Autodesk Fusion 360 part; units mm, degrees
note: some values were not read from the file. Set by a fixed rule: which sketch regions a step uses.
(part 2 of 3)
sketch "Sketch3" plane through (0, 0, -2) normal (0, 0, -1) x (1, 0, 0)
  line L0 (37.09, -0.4341) -> (37.09, -14.4986)
  arc A0 (32.09, -19.4986) -> (37.09, -14.4986) centre (32.09, -14.4986) ccw
  line L1 (32.09, -19.4986) -> (5.9194, -19.4986)
  arc A1 (0.9194, -14.4986) -> (5.9194, -19.4986) centre (5.9194, -14.4986) ccw
  line L2 (0.9194, -14.4986) -> (0.9194, -0.4341)
  line L3 (0.9194, -0.4341) -> (0.0951, -0.4341)
  line L4 (0.0951, -0.4341) -> (0.0951, -148.071)
  line L5 (0.0951, -148.071) -> (76.2953, -148.071)
  line L6 (76.2953, -148.071) -> (76.2953, -75.8337)
  line L7 (76.2953, -75.8337) -> (61.902, -75.8337)
  arc A2 (56.902, -70.8337) -> (61.902, -75.8337) centre (61.902, -70.8337) ccw
  line L8 (56.902, -70.8337) -> (56.902, -44.1838)
  arc A3 (61.902, -39.1838) -> (56.902, -44.1838) centre (61.902, -44.1838) ccw
  line L9 (61.902, -39.1838) -> (76.2953, -39.1838)
  line L10 (76.2953, -39.1838) -> (76.2953, -36.6991)
  line L11 (76.2953, -36.6991) -> (61.902, -36.6991)
  arc A4 (56.902, -31.6991) -> (61.902, -36.6991) centre (61.902, -31.6991) ccw
  line L12 (56.902, -31.6991) -> (56.902, -6.8092)
  arc A5 (61.902, -1.8092) -> (56.902, -6.8092) centre (61.902, -6.8092) ccw
  line L13 (61.902, -1.8092) -> (76.2953, -1.8092)
  line L14 (76.2953, -1.8092) -> (76.2953, -0.4341)
  line L15 (76.2953, -0.4341) -> (37.09, -0.4341)
  line L16 (40.7197, -3.5609) -> (40.7197, -1.96)
  line L17 (40.7197, -1.96) -> (54.719, -1.96)
  line L18 (54.719, -1.96) -> (54.719, -3.5609)
  line L19 (54.719, -3.5609) -> (55.5198, -3.5609)
  line L20 (55.5198, -3.5609) -> (55.5198, -16.3601)
  line L21 (55.5198, -16.3601) -> (54.719, -16.3601)
  line L22 (54.719, -16.3601) -> (54.719, -17.9595)
  line L23 (54.719, -17.9595) -> (40.7197, -17.9595)
  line L24 (40.7197, -17.9595) -> (40.7197, -16.3601)
  line L25 (40.7197, -16.3601) -> (39.9189, -16.3601)
  line L26 (39.9189, -16.3601) -> (39.9189, -3.5609)
  line L27 (39.9189, -3.5609) -> (40.7197, -3.5609)
  line L28 (2.6197, -79.7609) -> (2.6197, -78.1602)
  line L29 (2.6197, -78.1602) -> (16.6192, -78.1602)
  line L30 (16.6192, -78.1602) -> (16.6192, -79.7609)
  line L31 (16.6192, -79.7609) -> (17.4198, -79.7609)
  line L32 (17.4198, -79.7609) -> (17.4198, -92.5601)
  line L33 (17.4198, -92.5601) -> (16.6192, -92.5601)
  line L34 (16.6192, -92.5601) -> (16.6192, -94.1594)
  line L35 (16.6192, -94.1594) -> (2.6196, -94.1594)
  line L36 (2.6197, -94.1594) -> (2.6197, -92.5601)
  line L37 (2.6197, -92.5601) -> (1.819, -92.5601)
  line L38 (1.819, -92.5601) -> (1.819, -79.7609)
  line L39 (1.819, -79.7609) -> (2.6197, -79.7609)
  line L40 (21.6697, -22.6109) -> (21.6697, -21.01)
  line L41 (21.6697, -21.01) -> (35.669, -21.01)
  line L42 (35.669, -21.01) -> (35.669, -22.6109)
  line L43 (35.669, -22.6109) -> (36.4698, -22.6109)
  line L44 (36.4698, -22.6109) -> (36.4698, -35.4101)
  line L45 (36.4698, -35.4101) -> (35.669, -35.4101)
  line L46 (35.669, -35.4101) -> (35.669, -37.0094)
  line L47 (35.669, -37.0094) -> (21.6697, -37.0094)
  line L48 (21.6697, -37.0094) -> (21.6697, -35.4101)
  line L49 (21.6697, -35.4101) -> (20.869, -35.4101)
  line L50 (20.869, -35.4101) -> (20.869, -22.6109)
  line L51 (20.869, -22.6109) -> (21.6697, -22.6109)
  line L52 (40.7197, -41.6609) -> (40.7197, -40.0602)
  line L53 (40.7197, -40.0602) -> (54.719, -40.0602)
  line L54 (54.719, -40.0602) -> (54.719, -41.6609)
  line L55 (54.719, -41.6609) -> (55.5198, -41.6609)
  line L56 (55.5198, -41.6609) -> (55.5198, -54.4601)
  line L57 (55.5198, -54.4601) -> (54.719, -54.4601)
  line L58 (54.719, -54.4601) -> (54.719, -56.0594)
  line L59 (54.719, -56.0594) -> (40.7197, -56.0594)
  line L60 (40.7197, -56.0594) -> (40.7197, -54.4601)
  line L61 (40.7197, -54.4601) -> (39.9189, -54.4601)
  line L62 (39.9189, -54.4601) -> (39.9189, -41.6609)
  line L63 (39.9189, -41.6609) -> (40.7197, -41.6609)
  line L64 (40.7197, -22.6109) -> (40.7197, -21.01)
  line L65 (40.7197, -21.01) -> (54.719, -21.01)
  line L66 (54.719, -21.01) -> (54.719, -22.6109)
  line L67 (54.719, -22.6109) -> (55.5198, -22.6109)
  line L68 (55.5198, -22.6109) -> (55.5198, -35.4101)
  line L69 (55.5198, -35.4101) -> (54.719, -35.4101)
  line L70 (54.719, -35.4101) -> (54.719, -37.0094)
  line L71 (54.719, -37.0094) -> (40.7197, -37.0094)
  line L72 (40.7197, -37.0094) -> (40.7197, -35.4101)
  line L73 (40.7197, -35.4101) -> (39.9189, -35.4101)
  line L74 (39.9189, -35.4101) -> (39.9189, -22.6109)
  line L75 (39.9189, -22.6109) -> (40.7197, -22.6109)
  line L76 (40.7197, -60.7109) -> (40.7197, -59.1102)
  line L77 (40.7197, -59.1102) -> (54.719, -59.1102)
  line L78 (54.719, -59.1102) -> (54.719, -60.7109)
  line L79 (54.719, -60.7109) -> (55.5198, -60.7109)
  line L80 (55.5198, -60.7109) -> (55.5198, -73.5101)
  line L81 (55.5198, -73.5101) -> (54.719, -73.5101)
  line L82 (54.719, -73.5101) -> (54.719, -75.1094)
  line L83 (54.719, -75.1094) -> (40.7197, -75.1094)
  line L84 (40.7197, -75.1094) -> (40.7197, -73.5101)
  line L85 (40.7197, -73.5101) -> (39.9189, -73.5101)
  line L86 (39.9189, -73.5101) -> (39.9189, -60.7109)
  line L87 (39.9189, -60.7109) -> (40.7197, -60.7109)
  line L88 (21.6697, -41.6609) -> (21.6697, -40.0602)
  line L89 (21.6697, -40.0602) -> (35.669, -40.0602)
  line L90 (35.669, -40.0602) -> (35.669, -41.6609)
  line L91 (35.669, -41.6609) -> (36.4698, -41.6609)
  line L92 (36.4698, -41.6609) -> (36.4698, -54.4601)
  line L93 (36.4698, -54.4601) -> (35.669, -54.4601)
  line L94 (35.669, -54.4601) -> (35.669, -56.0594)
  line L95 (35.669, -56.0594) -> (21.6697, -56.0594)
  line L96 (21.6697, -56.0594) -> (21.6697, -54.4601)
  line L97 (21.6697, -54.4601) -> (20.869, -54.4601)
  line L98 (20.869, -54.4601) -> (20.869, -41.6609)
  line L99 (20.869, -41.6609) -> (21.6697, -41.6609)
  line L100 (2.6197, -41.6609) -> (2.6197, -40.0602)
  line L101 (2.6197, -40.0602) -> (16.6192, -40.0602)
  line L102 (16.6192, -40.0602) -> (16.6192, -41.6609)
  line L103 (16.6192, -41.6609) -> (17.4198, -41.6609)
  line L104 (17.4198, -41.6609) -> (17.4198, -54.4601)
  line L105 (17.4198, -54.4601) -> (16.6192, -54.4601)
  line L106 (16.6192, -54.4601) -> (16.6192, -56.0594)
  line L107 (16.6192, -56.0594) -> (2.6196, -56.0594)
  line L108 (2.6197, -56.0594) -> (2.6197, -54.4601)
  line L109 (2.6197, -54.4601) -> (1.819, -54.4601)
  line L110 (1.819, -54.4601) -> (1.819, -41.6609)
  line L111 (1.819, -41.6609) -> (2.6197, -41.6609)
  line L112 (2.6197, -22.6109) -> (2.6197, -21.01)
  line L113 (2.6197, -21.01) -> (16.6192, -21.01)
  line L114 (16.6192, -21.01) -> (16.6192, -22.6109)
  line L115 (16.6192, -22.6109) -> (17.4198, -22.6109)
  line L116 (17.4198, -22.6109) -> (17.4198, -35.4101)
  line L117 (17.4198, -35.4101) -> (16.6192, -35.4101)
  line L118 (16.6192, -35.4101) -> (16.6192, -37.0094)
  line L119 (16.6192, -37.0094) -> (2.6196, -37.0094)
  line L120 (2.6197, -37.0094) -> (2.6197, -35.4101)
  line L121 (2.6197, -35.4101) -> (1.819, -35.4101)
  line L122 (1.819, -35.4101) -> (1.819, -22.6109)
  line L123 (1.819, -22.6109) -> (2.6197, -22.6109)
  line L124 (40.7197, -79.7609) -> (40.7197, -78.1602)
  line L125 (40.7197, -78.1602) -> (54.719, -78.1602)
  line L126 (54.719, -78.1602) -> (54.719, -79.7609)
  line L127 (54.719, -79.7609) -> (55.5198, -79.7609)
  line L128 (55.5198, -79.7609) -> (55.5198, -92.5601)
  line L129 (55.5198, -92.5601) -> (54.719, -92.5601)
  line L130 (54.719, -92.5601) -> (54.719, -94.1594)
  line L131 (54.719, -94.1594) -> (40.7197, -94.1594)
  line L132 (40.7197, -94.1594) -> (40.7197, -92.5601)
  line L133 (40.7197, -92.5601) -> (39.9189, -92.5601)
  line L134 (39.9189, -92.5601) -> (39.9189, -79.7609)
  line L135 (39.9189, -79.7609) -> (40.7197, -79.7609)
  line L136 (59.7697, -79.7609) -> (59.7697, -78.1602)
  line L137 (59.7697, -78.1602) -> (73.769, -78.1602)
  line L138 (73.769, -78.1602) -> (73.769, -79.7609)
  line L139 (73.769, -79.7609) -> (74.5698, -79.7609)
  line L140 (74.5698, -79.7609) -> (74.5698, -92.5601)
  line L141 (74.5698, -92.5601) -> (73.769, -92.5601)
  line L142 (73.769, -92.5601) -> (73.769, -94.1594)
  line L143 (73.769, -94.1594) -> (59.7697, -94.1594)
  line L144 (59.7697, -94.1594) -> (59.7697, -92.5601)
  line L145 (59.7697, -92.5601) -> (58.9689, -92.5601)
  line L146 (58.9689, -92.5601) -> (58.9689, -79.7609)
  line L147 (58.9689, -79.7609) -> (59.7697, -79.7609)
  line L148 (2.6197, -60.7109) -> (2.6197, -59.1102)
  line L149 (2.6197, -59.1102) -> (16.6192, -59.1102)
  line L150 (16.6192, -59.1102) -> (16.6192, -60.7109)
  line L151 (16.6192, -60.7109) -> (17.4198, -60.7109)
  line L152 (17.4198, -60.7109) -> (17.4198, -73.5101)
  line L153 (17.4198, -73.5101) -> (16.6192, -73.5101)
  line L154 (16.6192, -73.5101) -> (16.6192, -75.1094)
  line L155 (16.6192, -75.1094) -> (2.6196, -75.1094)
  line L156 (2.6197, -75.1094) -> (2.6197, -73.5101)
  line L157 (2.6197, -73.5101) -> (1.819, -73.5101)
  line L158 (1.819, -73.5101) -> (1.819, -60.7109)
  line L159 (1.819, -60.7109) -> (2.6197, -60.7109)
  line L160 (59.7697, -117.861) -> (59.7697, -116.26)
  line L161 (59.7697, -116.26) -> (73.769, -116.26)
  line L162 (73.769, -116.26) -> (73.769, -117.861)
  line L163 (73.769, -117.861) -> (74.5698, -117.861)
  line L164 (74.5698, -117.861) -> (74.5698, -130.66)
  line L165 (74.5698, -130.66) -> (73.769, -130.66)
  line L166 (73.769, -130.66) -> (73.769, -132.259)
  line L167 (73.769, -132.259) -> (59.7697, -132.259)
  line L168 (59.7697, -132.259) -> (59.7697, -130.66)
  line L169 (59.7697, -130.66) -> (58.9689, -130.66)
  line L170 (58.9689, -130.66) -> (58.9689, -117.861)
  line L171 (58.9689, -117.861) -> (59.7697, -117.861)
  line L172 (21.6697, -79.7609) -> (21.6697, -78.1602)
  line L173 (21.6697, -78.1602) -> (35.669, -78.1602)
  line L174 (35.669, -78.1602) -> (35.669, -79.7609)
  line L175 (35.669, -79.7609) -> (36.4698, -79.7609)
  line L176 (36.4698, -79.7609) -> (36.4698, -92.5601)
  line L177 (36.4698, -92.5601) -> (35.669, -92.5601)
  line L178 (35.669, -92.5601) -> (35.669, -94.1594)
  line L179 (35.669, -94.1594) -> (21.6697, -94.1594)
  line L180 (21.6697, -94.1594) -> (21.6697, -92.5601)
  line L181 (21.6697, -92.5601) -> (20.869, -92.5601)
  line L182 (20.869, -92.5601) -> (20.869, -79.7609)
  line L183 (20.869, -79.7609) -> (21.6697, -79.7609)
  line L184 (21.6697, -60.7109) -> (21.6697, -59.1102)
  line L185 (21.6697, -59.1102) -> (35.669, -59.1102)
  line L186 (35.669, -59.1102) -> (35.669, -60.7109)
  line L187 (35.669, -60.7109) -> (36.4698, -60.7109)
  line L188 (36.4698, -60.7109) -> (36.4698, -73.5101)
  line L189 (36.4698, -73.5101) -> (35.669, -73.5101)
  line L190 (35.669, -73.5101) -> (35.669, -75.1094)
  line L191 (35.669, -75.1094) -> (21.6697, -75.1094)
  line L192 (21.6697, -75.1094) -> (21.6697, -73.5101)
  line L193 (21.6697, -73.5101) -> (20.869, -73.5101)
  line L194 (20.869, -73.5101) -> (20.869, -60.7109)
  line L195 (20.869, -60.7109) -> (21.6697, -60.7109)
  line L196 (47.7193, -17.9595) -> (47.7193, -1.96)
  line L197 (55.5198, -9.9605) -> (39.9189, -9.9605)
  line L198 (76.2953, -0.4341) -> (76.2953, 14.2999)
  line L199 (0.0951, -0.4341) -> (0.0951, 14.2999)
  line L200 (0.0951, 14.2999) -> (76.2953, 14.2999)
  line L201 (0.0951, -148.071) -> (0.0951, -158.6)
  line L202 (76.2953, -148.071) -> (76.2953, -158.6)
  line L203 (58.9689, -124.2605) -> (74.5698, -124.2605)
  line L204 (76.2953, -158.6) -> (76.2953, -163.6)
  line L205 (0.0951, -158.6) -> (0.0951, -163.6)
  line L206 (0.0951, -163.6) -> (76.2953, -163.6)
  line L207 (37.09, -0.4341) -> (0.0951, -0.4341)
  dimension "d38" = 14.734
  dimension "d39" = 14.734
  dimension "d42" = 5
  dimension "d43" = 5
  dimension "d44" = 177.8999
  constraint midpoint L23 L196.start
  constraint midpoint L17 L196.end
  constraint midpoint L20 L197.start
  constraint midpoint L26 L197.end
  constraint coincident L14.end L15.start
  constraint perpendicular L15 L198
  constraint coincident L3.end L4.start
  constraint perpendicular L3 L199
  constraint coincident L4.end L5.start
  constraint perpendicular L5 L201
  constraint coincident L5.end L6.start
  constraint perpendicular L5 L202
  constraint midpoint L170 L203.start
  constraint midpoint L164 L203.end
  constraint coincident L0.start L15.end
  measures "d38" distance of L14.end L198.end
  measures "d39" distance of L3.end L199.end
  measures "d42" distance of L202.end L204.end
  measures "d43" distance of L201.end L205.end
  measures "d44" distance of L200 L206
extrude "Extrude19" add sketch "Sketch3" against normal blind 3 contours L3 L15 L198 L199 L200 L207 | L5 L201 L202 L204 L205 L206 bodies 1 2
sketch "Sketch4" plane through (0, 0, -2) normal (0, 0, -1) x (1, 0, 0)
  line L0 (37.09, -0.4341) -> (37.09, -14.4986)
  arc A0 (32.09, -19.4986) -> (37.09, -14.4986) centre (32.09, -14.4986) ccw
  line L1 (32.09, -19.4986) -> (5.9194, -19.4986)
  arc A1 (0.9194, -14.4986) -> (5.9194, -19.4986) centre (5.9194, -14.4986) ccw
  line L2 (0.9194, -14.4986) -> (0.9194, -0.4341)
  line L3 (0.9194, -0.4341) -> (37.09, -0.4341)
  line L4 (76.2953, -1.8092) -> (76.2953, 14.2999)
  line L5 (76.2953, 14.2999) -> (0.0951, 14.2999)
  line L6 (0.0951, 14.2999) -> (0.0951, -163.6)
  line L7 (0.0951, -163.6) -> (76.2953, -163.6)
  line L8 (76.2953, -163.6) -> (76.2953, -75.8337)
  line L9 (76.2953, -75.8337) -> (61.902, -75.8337)
  arc A2 (56.902, -70.8337) -> (61.902, -75.8337) centre (61.902, -70.8337) ccw
  line L10 (56.902, -70.8337) -> (56.902, -44.1838)
  arc A3 (61.902, -39.1838) -> (56.902, -44.1838) centre (61.902, -44.1838) ccw
  line L11 (61.902, -39.1838) -> (76.2953, -39.1838)
  line L12 (76.2953, -39.1838) -> (76.2953, -36.6991)
  line L13 (76.2953, -36.6991) -> (61.902, -36.6991)
  arc A4 (56.902, -31.6991) -> (61.902, -36.6991) centre (61.902, -31.6991) ccw
  line L14 (56.902, -31.6991) -> (56.902, -6.8092)
  arc A5 (61.902, -1.8092) -> (56.902, -6.8092) centre (61.902, -6.8092) ccw
  line L15 (61.902, -1.8092) -> (76.2953, -1.8092)
  line L16 (40.7197, -3.5609) -> (40.7197, -1.96)
  line L17 (40.7197, -1.96) -> (54.719, -1.96)
  line L18 (54.719, -1.96) -> (54.719, -3.5609)
  line L19 (54.719, -3.5609) -> (55.5198, -3.5609)
  line L20 (55.5198, -3.5609) -> (55.5198, -16.3601)
  line L21 (55.5198, -16.3601) -> (54.719, -16.3601)
  line L22 (54.719, -16.3601) -> (54.719, -17.9595)
  line L23 (54.719, -17.9595) -> (40.7197, -17.9595)
  line L24 (40.7197, -17.9595) -> (40.7197, -16.3601)
  line L25 (40.7197, -16.3601) -> (39.9189, -16.3601)
  line L26 (39.9189, -16.3601) -> (39.9189, -3.5609)
  line L27 (39.9189, -3.5609) -> (40.7197, -3.5609)
  line L28 (2.6197, -79.7609) -> (2.6197, -78.1602)
  line L29 (2.6197, -78.1602) -> (16.6192, -78.1602)
  line L30 (16.6192, -78.1602) -> (16.6192, -79.7609)
  line L31 (16.6192, -79.7609) -> (17.4198, -79.7609)
  line L32 (17.4198, -79.7609) -> (17.4198, -92.5601)
  line L33 (17.4198, -92.5601) -> (16.6192, -92.5601)
  line L34 (16.6192, -92.5601) -> (16.6192, -94.1594)
  line L35 (16.6192, -94.1594) -> (2.6196, -94.1594)
  line L36 (2.6197, -94.1594) -> (2.6197, -92.5601)
  line L37 (2.6197, -92.5601) -> (1.819, -92.5601)
  line L38 (1.819, -92.5601) -> (1.819, -79.7609)
  line L39 (1.819, -79.7609) -> (2.6197, -79.7609)
  line L40 (21.6697, -22.6109) -> (21.6697, -21.01)
  line L41 (21.6697, -21.01) -> (35.669, -21.01)
  line L42 (35.669, -21.01) -> (35.669, -22.6109)
  line L43 (35.669, -22.6109) -> (36.4698, -22.6109)
  line L44 (36.4698, -22.6109) -> (36.4698, -35.4101)
  line L45 (36.4698, -35.4101) -> (35.669, -35.4101)
  line L46 (35.669, -35.4101) -> (35.669, -37.0094)
  line L47 (35.669, -37.0094) -> (21.6697, -37.0094)
  line L48 (21.6697, -37.0094) -> (21.6697, -35.4101)
  line L49 (21.6697, -35.4101) -> (20.869, -35.4101)
  line L50 (20.869, -35.4101) -> (20.869, -22.6109)
  line L51 (20.869, -22.6109) -> (21.6697, -22.6109)
  line L52 (40.7197, -41.6609) -> (40.7197, -40.0602)
  line L53 (40.7197, -40.0602) -> (54.719, -40.0602)
  line L54 (54.719, -40.0602) -> (54.719, -41.6609)
  line L55 (54.719, -41.6609) -> (55.5198, -41.6609)
  line L56 (55.5198, -41.6609) -> (55.5198, -54.4601)
  line L57 (55.5198, -54.4601) -> (54.719, -54.4601)
  line L58 (54.719, -54.4601) -> (54.719, -56.0594)
  line L59 (54.719, -56.0594) -> (40.7197, -56.0594)
  line L60 (40.7197, -56.0594) -> (40.7197, -54.4601)
  line L61 (40.7197, -54.4601) -> (39.9189, -54.4601)
  line L62 (39.9189, -54.4601) -> (39.9189, -41.6609)
  line L63 (39.9189, -41.6609) -> (40.7197, -41.6609)
  line L64 (40.7197, -22.6109) -> (40.7197, -21.01)
  line L65 (40.7197, -21.01) -> (54.719, -21.01)
  line L66 (54.719, -21.01) -> (54.719, -22.6109)
  line L67 (54.719, -22.6109) -> (55.5198, -22.6109)
  line L68 (55.5198, -22.6109) -> (55.5198, -35.4101)
  line L69 (55.5198, -35.4101) -> (54.719, -35.4101)
  line L70 (54.719, -35.4101) -> (54.719, -37.0094)
  line L71 (54.719, -37.0094) -> (40.7197, -37.0094)
  line L72 (40.7197, -37.0094) -> (40.7197, -35.4101)
  line L73 (40.7197, -35.4101) -> (39.9189, -35.4101)
  line L74 (39.9189, -35.4101) -> (39.9189, -22.6109)
  line L75 (39.9189, -22.6109) -> (40.7197, -22.6109)
  line L76 (40.7197, -60.7109) -> (40.7197, -59.1102)
  line L77 (40.7197, -59.1102) -> (54.719, -59.1102)
  line L78 (54.719, -59.1102) -> (54.719, -60.7109)
  line L79 (54.719, -60.7109) -> (55.5198, -60.7109)
  line L80 (55.5198, -60.7109) -> (55.5198, -73.5101)
  line L81 (55.5198, -73.5101) -> (54.719, -73.5101)
  line L82 (54.719, -73.5101) -> (54.719, -75.1094)
  line L83 (54.719, -75.1094) -> (40.7197, -75.1094)
  line L84 (40.7197, -75.1094) -> (40.7197, -73.5101)
  line L85 (40.7197, -73.5101) -> (39.9189, -73.5101)
  line L86 (39.9189, -73.5101) -> (39.9189, -60.7109)
  line L87 (39.9189, -60.7109) -> (40.7197, -60.7109)
  line L88 (21.6697, -41.6609) -> (21.6697, -40.0602)
  line L89 (21.6697, -40.0602) -> (35.669, -40.0602)
  line L90 (35.669, -40.0602) -> (35.669, -41.6609)
  line L91 (35.669, -41.6609) -> (36.4698, -41.6609)
  line L92 (36.4698, -41.6609) -> (36.4698, -54.4601)
  line L93 (36.4698, -54.4601) -> (35.669, -54.4601)
  line L94 (35.669, -54.4601) -> (35.669, -56.0594)
  line L95 (35.669, -56.0594) -> (21.6697, -56.0594)
  line L96 (21.6697, -56.0594) -> (21.6697, -54.4601)
  line L97 (21.6697, -54.4601) -> (20.869, -54.4601)
  line L98 (20.869, -54.4601) -> (20.869, -41.6609)
  line L99 (20.869, -41.6609) -> (21.6697, -41.6609)
  line L100 (2.6197, -41.6609) -> (2.6197, -40.0602)
  line L101 (2.6197, -40.0602) -> (16.6192, -40.0602)
  line L102 (16.6192, -40.0602) -> (16.6192, -41.6609)
  line L103 (16.6192, -41.6609) -> (17.4198, -41.6609)
  line L104 (17.4198, -41.6609) -> (17.4198, -54.4601)
  line L105 (17.4198, -54.4601) -> (16.6192, -54.4601)
  line L106 (16.6192, -54.4601) -> (16.6192, -56.0594)
  line L107 (16.6192, -56.0594) -> (2.6196, -56.0594)
  line L108 (2.6197, -56.0594) -> (2.6197, -54.4601)
  line L109 (2.6197, -54.4601) -> (1.819, -54.4601)
  line L110 (1.819, -54.4601) -> (1.819, -41.6609)
  line L111 (1.819, -41.6609) -> (2.6197, -41.6609)
  line L112 (2.6197, -22.6109) -> (2.6197, -21.01)
  line L113 (2.6197, -21.01) -> (16.6192, -21.01)
  line L114 (16.6192, -21.01) -> (16.6192, -22.6109)
  line L115 (16.6192, -22.6109) -> (17.4198, -22.6109)
  line L116 (17.4198, -22.6109) -> (17.4198, -35.4101)
  line L117 (17.4198, -35.4101) -> (16.6192, -35.4101)
  line L118 (16.6192, -35.4101) -> (16.6192, -37.0094)
  line L119 (16.6192, -37.0094) -> (2.6196, -37.0094)
  line L120 (2.6197, -37.0094) -> (2.6197, -35.4101)
  line L121 (2.6197, -35.4101) -> (1.819, -35.4101)
  line L122 (1.819, -35.4101) -> (1.819, -22.6109)
  line L123 (1.819, -22.6109) -> (2.6197, -22.6109)
  line L124 (40.7197, -79.7609) -> (40.7197, -78.1602)
  line L125 (40.7197, -78.1602) -> (54.719, -78.1602)
  line L126 (54.719, -78.1602) -> (54.719, -79.7609)
  line L127 (54.719, -79.7609) -> (55.5198, -79.7609)
  line L128 (55.5198, -79.7609) -> (55.5198, -92.5601)
  line L129 (55.5198, -92.5601) -> (54.719, -92.5601)
  line L130 (54.719, -92.5601) -> (54.719, -94.1594)
  line L131 (54.719, -94.1594) -> (40.7197, -94.1594)
  line L132 (40.7197, -94.1594) -> (40.7197, -92.5601)
  line L133 (40.7197, -92.5601) -> (39.9189, -92.5601)
  line L134 (39.9189, -92.5601) -> (39.9189, -79.7609)
  line L135 (39.9189, -79.7609) -> (40.7197, -79.7609)
  line L136 (59.7697, -79.7609) -> (59.7697, -78.1602)
  line L137 (59.7697, -78.1602) -> (73.769, -78.1602)
  line L138 (73.769, -78.1602) -> (73.769, -79.7609)
  line L139 (73.769, -79.7609) -> (74.5698, -79.7609)
  line L140 (74.5698, -79.7609) -> (74.5698, -92.5601)
  line L141 (74.5698, -92.5601) -> (73.769, -92.5601)
  line L142 (73.769, -92.5601) -> (73.769, -94.1594)
  line L143 (73.769, -94.1594) -> (59.7697, -94.1594)
  line L144 (59.7697, -94.1594) -> (59.7697, -92.5601)
  line L145 (59.7697, -92.5601) -> (58.9689, -92.5601)
  line L146 (58.9689, -92.5601) -> (58.9689, -79.7609)
  line L147 (58.9689, -79.7609) -> (59.7697, -79.7609)
  line L148 (2.6197, -60.7109) -> (2.6197, -59.1102)
  line L149 (2.6197, -59.1102) -> (16.6192, -59.1102)
  line L150 (16.6192, -59.1102) -> (16.6192, -60.7109)
  line L151 (16.6192, -60.7109) -> (17.4198, -60.7109)
  line L152 (17.4198, -60.7109) -> (17.4198, -73.5101)
  line L153 (17.4198, -73.5101) -> (16.6192, -73.5101)
  line L154 (16.6192, -73.5101) -> (16.6192, -75.1094)
  line L155 (16.6192, -75.1094) -> (2.6196, -75.1094)
  line L156 (2.6197, -75.1094) -> (2.6197, -73.5101)
  line L157 (2.6197, -73.5101) -> (1.819, -73.5101)
  line L158 (1.819, -73.5101) -> (1.819, -60.7109)
  line L159 (1.819, -60.7109) -> (2.6197, -60.7109)
  line L160 (59.7697, -117.861) -> (59.7697, -116.26)
  line L161 (59.7697, -116.26) -> (73.769, -116.26)
  line L162 (73.769, -116.26) -> (73.769, -117.861)
  line L163 (73.769, -117.861) -> (74.5698, -117.861)
  line L164 (74.5698, -117.861) -> (74.5698, -130.66)
  line L165 (74.5698, -130.66) -> (73.769, -130.66)
  line L166 (73.769, -130.66) -> (73.769, -132.259)
  line L167 (73.769, -132.259) -> (59.7697, -132.259)
  line L168 (59.7697, -132.259) -> (59.7697, -130.66)
  line L169 (59.7697, -130.66) -> (58.9689, -130.66)
  line L170 (58.9689, -130.66) -> (58.9689, -117.861)
  line L171 (58.9689, -117.861) -> (59.7697, -117.861)
  line L172 (21.6697, -79.7609) -> (21.6697, -78.1602)
  line L173 (21.6697, -78.1602) -> (35.669, -78.1602)
  line L174 (35.669, -78.1602) -> (35.669, -79.7609)
  line L175 (35.669, -79.7609) -> (36.4698, -79.7609)
  line L176 (36.4698, -79.7609) -> (36.4698, -92.5601)
  line L177 (36.4698, -92.5601) -> (35.669, -92.5601)
  line L178 (35.669, -92.5601) -> (35.669, -94.1594)
  line L179 (35.669, -94.1594) -> (21.6697, -94.1594)
  line L180 (21.6697, -94.1594) -> (21.6697, -92.5601)
  line L181 (21.6697, -92.5601) -> (20.869, -92.5601)
  line L182 (20.869, -92.5601) -> (20.869, -79.7609)
  line L183 (20.869, -79.7609) -> (21.6697, -79.7609)
  line L184 (21.6697, -60.7109) -> (21.6697, -59.1102)
  line L185 (21.6697, -59.1102) -> (35.669, -59.1102)
  line L186 (35.669, -59.1102) -> (35.669, -60.7109)
  line L187 (35.669, -60.7109) -> (36.4698, -60.7109)
  line L188 (36.4698, -60.7109) -> (36.4698, -73.5101)
  line L189 (36.4698, -73.5101) -> (35.669, -73.5101)
  line L190 (35.669, -73.5101) -> (35.669, -75.1094)
  line L191 (35.669, -75.1094) -> (21.6697, -75.1094)
  line L192 (21.6697, -75.1094) -> (21.6697, -73.5101)
  line L193 (21.6697, -73.5101) -> (20.869, -73.5101)
  line L194 (20.869, -73.5101) -> (20.869, -60.7109)
  line L195 (20.869, -60.7109) -> (21.6697, -60.7109)
  line L196 (66.7694, -132.259) -> (66.7694, -116.26)
  line L197 (76.2953, -163.6) -> (87.4343, -163.6)
  line L198 (76.2953, 14.2999) -> (87.4343, 14.2999)
  line L199 (87.4343, -163.6) -> (87.4343, 14.2999)
  line L200 (76.2953, 14.2999) -> (76.2953, -163.6)
  line L201 (9.6194, -78.1602) -> (9.6194, -103.261)
  line L202 (0.0951, -163.6) -> (-11.1659, -163.6)
  line L203 (0.0951, 14.2999) -> (-11.1659, 14.2999)
  line L204 (-11.1659, 14.2999) -> (-11.1659, -163.6)
  dimension "d47" = 11.139
  dimension "d48" = 11.139
  dimension "d49" = 11.261
  dimension "d50" = 11.261
  constraint midpoint L167 L196.start
  constraint midpoint L161 L196.end
  constraint coincident L7.end L8.start
  constraint perpendicular L8 L197
  constraint coincident L4.end L5.start
  constraint perpendicular L4 L198
  constraint midpoint L29 L201.start
  constraint perpendicular L29 L201
  constraint coincident L6.end L7.start
  constraint perpendicular L6 L202
  constraint coincident L5.end L6.start
  constraint perpendicular L6 L203
  measures "d47" distance of L7.end L197.end
  measures "d48" distance of L4.end L198.end
  measures "d49" distance of L6.end L202.end
  measures "d50" distance of L5.end L203.end
extrude "Extrude20" add sketch "Sketch4" against normal blind 3 contours L4 L8 L12 L197 L198 L199 L200 | L6 L202 L203 L204 bodies 1
sketch "Sketch5" plane through (0, 0, 1) normal (0, 0, 1) x (-1, 0, 0)
  line L0 (-21.6697, -74.1094) -> (-35.669, -74.1094)
  line L1 (-35.669, -74.1094) -> (-35.669, -73.5101)
  line L2 (-35.669, -73.5101) -> (-36.4698, -73.5101)
  line L3 (-36.4698, -73.5101) -> (-36.4698, -60.7109)
  line L4 (-36.4698, -60.7109) -> (-35.669, -60.7109)
  line L5 (-35.669, -60.7109) -> (-35.669, -60.1102)
  line L6 (-35.669, -60.1102) -> (-21.6697, -60.1102)
  line L7 (-21.6697, -60.1102) -> (-21.6697, -60.7109)
  line L8 (-21.6697, -60.7109) -> (-20.869, -60.7109)
  line L9 (-20.869, -60.7109) -> (-20.869, -73.5101)
  line L10 (-20.869, -73.5101) -> (-21.6697, -73.5101)
  line L11 (-21.6697, -73.5101) -> (-21.6697, -74.1094)
  line L12 (-66.27, -35.585) -> (-69.07, -35.585)
  line L13 (-69.07, -35.585) -> (-69.07, -34.7597)
  line L14 (-69.07, -34.7597) -> (-72.3, -34.7597)
  line L15 (-72.3, -34.7597) -> (-72.3, -28.01)
  line L16 (-72.3, -28.01) -> (-69.07, -28.01)
  line L17 (-69.07, -28.01) -> (-69.07, -27.2852)
  line L18 (-69.07, -27.2852) -> (-73.1696, -27.2852)
  line L19 (-73.1696, -27.2852) -> (-73.1696, -26.4845)
  line L20 (-73.1696, -26.4845) -> (-73.769, -26.4845)
  line L21 (-73.769, -26.4845) -> (-73.769, -12.485)
  line L22 (-73.769, -12.485) -> (-73.1696, -12.485)
  line L23 (-73.1696, -12.485) -> (-73.1696, -11.6858)
  line L24 (-73.1696, -11.6858) -> (-69.07, -11.6858)
  line L25 (-69.07, -11.6858) -> (-69.07, -10.9595)
  line L26 (-69.07, -10.9595) -> (-72.3, -10.9595)
  line L27 (-72.3, -10.9595) -> (-72.3, -4.2099)
  line L28 (-72.3, -4.2099) -> (-69.07, -4.2099)
  line L29 (-69.07, -4.2099) -> (-69.07, -3.3858)
  line L30 (-69.07, -3.3858) -> (-66.27, -3.3858)
  line L31 (-66.27, -3.3858) -> (-66.27, -4.2099)
  line L32 (-66.27, -4.2099) -> (-59.9997, -4.2099)
  line L33 (-59.9997, -4.2099) -> (-59.9997, -5.9352)
  line L34 (-59.9997, -5.9352) -> (-58.7996, -5.9352)
  line L35 (-58.7996, -5.9352) -> (-58.7996, -9.2356)
  line L36 (-58.7996, -9.2356) -> (-59.9997, -9.2356)
  line L37 (-59.9997, -9.2356) -> (-59.9997, -10.9595)
  line L38 (-59.9997, -10.9595) -> (-64.4701, -10.9595)
  line L39 (-64.4701, -10.9595) -> (-64.4701, -11.6858)
  line L40 (-64.4701, -11.6858) -> (-60.3691, -11.6858)
  line L41 (-60.3691, -11.6858) -> (-60.3691, -12.485)
  line L42 (-60.3691, -12.485) -> (-59.7697, -12.485)
  line L43 (-59.7697, -12.485) -> (-59.7697, -26.4845)
  line L44 (-59.7697, -26.4845) -> (-60.3691, -26.4845)
  line L45 (-60.3691, -26.4845) -> (-60.3691, -27.2852)
  line L46 (-60.3691, -27.2852) -> (-64.4701, -27.2852)
  line L47 (-64.4701, -27.2852) -> (-64.4701, -28.01)
  line L48 (-64.4701, -28.01) -> (-59.9997, -28.01)
  line L49 (-59.9997, -28.01) -> (-59.9997, -29.7353)
  line L50 (-59.9997, -29.7353) -> (-58.7996, -29.7353)
  line L51 (-58.7996, -29.7353) -> (-58.7996, -33.0357)
  line L52 (-58.7996, -33.0357) -> (-59.9997, -33.0357)
  line L53 (-59.9997, -33.0357) -> (-59.9997, -34.7597)
  line L54 (-59.9997, -34.7597) -> (-66.27, -34.7597)
  line L55 (-66.27, -34.7597) -> (-66.27, -35.585)
  line L56 (-21.6697, -93.1594) -> (-35.669, -93.1594)
  line L57 (-35.669, -93.1594) -> (-35.669, -92.5601)
  line L58 (-35.669, -92.5601) -> (-36.4698, -92.5601)
  line L59 (-36.4698, -92.5601) -> (-36.4698, -79.7609)
  line L60 (-36.4698, -79.7609) -> (-35.669, -79.7609)
  line L61 (-35.669, -79.7609) -> (-35.669, -79.1602)
  line L62 (-35.669, -79.1602) -> (-21.6697, -79.1602)
  line L63 (-21.6697, -79.1602) -> (-21.6697, -79.7609)
  line L64 (-21.6697, -79.7609) -> (-20.869, -79.7609)
  line L65 (-20.869, -79.7609) -> (-20.869, -92.5601)
  line L66 (-20.869, -92.5601) -> (-21.6697, -92.5601)
  line L67 (-21.6697, -92.5601) -> (-21.6697, -93.1594)
  line L68 (-59.7697, -131.259) -> (-73.769, -131.259)
  line L69 (-73.769, -131.259) -> (-73.769, -130.66)
  line L70 (-73.769, -130.66) -> (-74.5698, -130.66)
  line L71 (-74.5698, -130.66) -> (-74.5698, -117.861)
  line L72 (-74.5698, -117.861) -> (-73.769, -117.861)
  line L73 (-73.769, -117.861) -> (-73.769, -117.26)
  line L74 (-73.769, -117.26) -> (-59.7697, -117.26)
  line L75 (-59.7697, -117.26) -> (-59.7697, -117.861)
  line L76 (-59.7697, -117.861) -> (-58.9689, -117.861)
  line L77 (-58.9689, -117.861) -> (-58.9689, -130.66)
  line L78 (-58.9689, -130.66) -> (-59.7697, -130.66)
  line L79 (-59.7697, -130.66) -> (-59.7697, -131.259)
  line L80 (-66.27, -73.685) -> (-69.07, -73.685)
  line L81 (-69.07, -73.685) -> (-69.07, -72.8595)
  line L82 (-69.07, -72.8595) -> (-72.3, -72.8595)
  line L83 (-72.3, -72.8595) -> (-72.3, -66.1098)
  line L84 (-72.3, -66.1098) -> (-69.07, -66.1098)
  line L85 (-69.07, -66.1098) -> (-69.07, -65.3852)
  line L86 (-69.07, -65.3852) -> (-73.1696, -65.3852)
  line L87 (-73.1696, -65.3852) -> (-73.1696, -64.5844)
  line L88 (-73.1696, -64.5844) -> (-73.769, -64.5844)
  line L89 (-73.769, -64.5844) -> (-73.769, -50.5852)
  line L90 (-73.769, -50.5852) -> (-73.1696, -50.5852)
  line L91 (-73.1696, -50.5852) -> (-73.1696, -49.7858)
  line L92 (-73.1696, -49.7858) -> (-69.07, -49.7858)
  line L93 (-69.07, -49.7858) -> (-69.07, -49.0594)
  line L94 (-69.07, -49.0594) -> (-72.3, -49.0594)
  line L95 (-72.3, -49.0594) -> (-72.3, -42.31)
  line L96 (-72.3, -42.31) -> (-69.07, -42.31)
  line L97 (-69.07, -42.31) -> (-69.07, -41.486)
  line L98 (-69.07, -41.486) -> (-66.27, -41.486)
  line L99 (-66.27, -41.486) -> (-66.27, -42.31)
  line L100 (-66.27, -42.31) -> (-59.9997, -42.31)
  line L101 (-59.9997, -42.31) -> (-59.9997, -44.0351)
  line L102 (-59.9997, -44.0351) -> (-58.7996, -44.0351)
  line L103 (-58.7996, -44.0351) -> (-58.7996, -47.3357)
  line L104 (-58.7996, -47.3357) -> (-59.9997, -47.3357)
  line L105 (-59.9997, -47.3357) -> (-59.9997, -49.0594)
  line L106 (-59.9997, -49.0594) -> (-64.4701, -49.0594)
  line L107 (-64.4701, -49.0594) -> (-64.4701, -49.7858)
  line L108 (-64.4701, -49.7858) -> (-60.3691, -49.7858)
  line L109 (-60.3691, -49.7858) -> (-60.3691, -50.5852)
  line L110 (-60.3691, -50.5852) -> (-59.7697, -50.5852)
  line L111 (-59.7697, -50.5852) -> (-59.7697, -64.5844)
  line L112 (-59.7697, -64.5844) -> (-60.3691, -64.5844)
  line L113 (-60.3691, -64.5844) -> (-60.3691, -65.3852)
  line L114 (-60.3691, -65.3852) -> (-64.4701, -65.3852)
  line L115 (-64.4701, -65.3852) -> (-64.4701, -66.1098)
  line L116 (-64.4701, -66.1098) -> (-59.9997, -66.1098)
  line L117 (-59.9997, -66.1098) -> (-59.9997, -67.8353)
  line L118 (-59.9997, -67.8353) -> (-58.7996, -67.8353)
  line L119 (-58.7996, -67.8353) -> (-58.7996, -71.1359)
  line L120 (-58.7996, -71.1359) -> (-59.9997, -71.1359)
  line L121 (-59.9997, -71.1359) -> (-59.9997, -72.8595)
  line L122 (-59.9997, -72.8595) -> (-66.27, -72.8595)
  line L123 (-66.27, -72.8595) -> (-66.27, -73.685)
  line L124 (-2.6197, -74.1094) -> (-16.6192, -74.1094)
  line L125 (-16.6192, -74.1094) -> (-16.6192, -73.5101)
  line L126 (-16.6192, -73.5101) -> (-17.4198, -73.5101)
  line L127 (-17.4198, -73.5101) -> (-17.4198, -60.7109)
  line L128 (-17.4198, -60.7109) -> (-16.6192, -60.7109)
  line L129 (-16.6192, -60.7109) -> (-16.6192, -60.1102)
  line L130 (-16.6192, -60.1102) -> (-2.6196, -60.1102)
  line L131 (-2.6197, -60.1102) -> (-2.6197, -60.7109)
  line L132 (-2.6197, -60.7109) -> (-1.819, -60.7109)
  line L133 (-1.819, -60.7109) -> (-1.819, -73.5101)
  line L134 (-1.819, -73.5101) -> (-2.6197, -73.5101)
  line L135 (-2.6197, -73.5101) -> (-2.6197, -74.1094)
  line L136 (-59.7697, -93.1594) -> (-73.769, -93.1594)
  line L137 (-73.769, -93.1594) -> (-73.769, -92.5601)
  line L138 (-73.769, -92.5601) -> (-74.5698, -92.5601)
  line L139 (-74.5698, -92.5601) -> (-74.5698, -79.7609)
  line L140 (-74.5698, -79.7609) -> (-73.769, -79.7609)
  line L141 (-73.769, -79.7609) -> (-73.769, -79.1602)
  line L142 (-73.769, -79.1602) -> (-59.7697, -79.1602)
  line L143 (-59.7697, -79.1602) -> (-59.7697, -79.7609)
  line L144 (-59.7697, -79.7609) -> (-58.9689, -79.7609)
  line L145 (-58.9689, -79.7609) -> (-58.9689, -92.5601)
  line L146 (-58.9689, -92.5601) -> (-59.7697, -92.5601)
  line L147 (-59.7697, -92.5601) -> (-59.7697, -93.1594)
  line L148 (-40.7197, -93.1594) -> (-54.719, -93.1594)
  line L149 (-54.719, -93.1594) -> (-54.719, -92.5601)
  line L150 (-54.719, -92.5601) -> (-55.5198, -92.5601)
  line L151 (-55.5198, -92.5601) -> (-55.5198, -79.7609)
  line L152 (-55.5198, -79.7609) -> (-54.719, -79.7609)
  line L153 (-54.719, -79.7609) -> (-54.719, -79.1602)
  line L154 (-54.719, -79.1602) -> (-40.7197, -79.1602)
  line L155 (-40.7197, -79.1602) -> (-40.7197, -79.7609)
  line L156 (-40.7197, -79.7609) -> (-39.9189, -79.7609)
  line L157 (-39.9189, -79.7609) -> (-39.9189, -92.5601)
  line L158 (-39.9189, -92.5601) -> (-40.7197, -92.5601)
  line L159 (-40.7197, -92.5601) -> (-40.7197, -93.1594)
  line L160 (-2.6197, -36.0094) -> (-16.6192, -36.0094)
  line L161 (-16.6192, -36.0094) -> (-16.6192, -35.4101)
  line L162 (-16.6192, -35.4101) -> (-17.4198, -35.4101)
  line L163 (-17.4198, -35.4101) -> (-17.4198, -22.6109)
  line L164 (-17.4198, -22.6109) -> (-16.6192, -22.6109)
  line L165 (-16.6192, -22.6109) -> (-16.6192, -22.01)
  line L166 (-16.6192, -22.01) -> (-2.6196, -22.01)
  line L167 (-2.6197, -22.01) -> (-2.6197, -22.6109)
  line L168 (-2.6197, -22.6109) -> (-1.819, -22.6109)
  line L169 (-1.819, -22.6109) -> (-1.819, -35.4101)
  line L170 (-1.819, -35.4101) -> (-2.6197, -35.4101)
  line L171 (-2.6197, -35.4101) -> (-2.6197, -36.0094)
  line L172 (-2.6197, -55.0594) -> (-16.6192, -55.0594)
  line L173 (-16.6192, -55.0594) -> (-16.6192, -54.4601)
  line L174 (-16.6192, -54.4601) -> (-17.4198, -54.4601)
  line L175 (-17.4198, -54.4601) -> (-17.4198, -41.6609)
  line L176 (-17.4198, -41.6609) -> (-16.6192, -41.6609)
  line L177 (-16.6192, -41.6609) -> (-16.6192, -41.0602)
  line L178 (-16.6192, -41.0602) -> (-2.6196, -41.0602)
  line L179 (-2.6197, -41.0602) -> (-2.6197, -41.6609)
  line L180 (-2.6197, -41.6609) -> (-1.819, -41.6609)
  line L181 (-1.819, -41.6609) -> (-1.819, -54.4601)
  line L182 (-1.819, -54.4601) -> (-2.6197, -54.4601)
  line L183 (-2.6197, -54.4601) -> (-2.6197, -55.0594)
  line L184 (-21.6697, -55.0594) -> (-35.669, -55.0594)
  line L185 (-35.669, -55.0594) -> (-35.669, -54.4601)
  line L186 (-35.669, -54.4601) -> (-36.4698, -54.4601)
  line L187 (-36.4698, -54.4601) -> (-36.4698, -41.6609)
  line L188 (-36.4698, -41.6609) -> (-35.669, -41.6609)
  line L189 (-35.669, -41.6609) -> (-35.669, -41.0602)
  line L190 (-35.669, -41.0602) -> (-21.6697, -41.0602)
  line L191 (-21.6697, -41.0602) -> (-21.6697, -41.6609)
  line L192 (-21.6697, -41.6609) -> (-20.869, -41.6609)
  line L193 (-20.869, -41.6609) -> (-20.869, -54.4601)
  line L194 (-20.869, -54.4601) -> (-21.6697, -54.4601)
  line L195 (-21.6697, -54.4601) -> (-21.6697, -55.0594)
  line L196 (-40.7197, -74.1094) -> (-54.719, -74.1094)
  line L197 (-54.719, -74.1094) -> (-54.719, -73.5101)
  line L198 (-54.719, -73.5101) -> (-55.5198, -73.5101)
  line L199 (-55.5198, -73.5101) -> (-55.5198, -60.7109)
  line L200 (-55.5198, -60.7109) -> (-54.719, -60.7109)
  line L201 (-54.719, -60.7109) -> (-54.719, -60.1102)
  line L202 (-54.719, -60.1102) -> (-40.7197, -60.1102)
  line L203 (-40.7197, -60.1102) -> (-40.7197, -60.7109)
  line L204 (-40.7197, -60.7109) -> (-39.9189, -60.7109)
  line L205 (-39.9189, -60.7109) -> (-39.9189, -73.5101)
  line L206 (-39.9189, -73.5101) -> (-40.7197, -73.5101)
  line L207 (-40.7197, -73.5101) -> (-40.7197, -74.1094)
  line L208 (-12.1447, -16.9595) -> (-26.1441, -16.9595)
  line L209 (-26.1441, -16.9595) -> (-26.1441, -16.3601)
  line L210 (-26.1441, -16.3601) -> (-26.9448, -16.3601)
  line L211 (-26.9448, -16.3601) -> (-26.9448, -12.2604)
  line L212 (-26.9448, -12.2604) -> (-27.6696, -12.2604)
  line L213 (-27.6696, -12.2604) -> (-27.6696, -15.4905)
  line L214 (-27.6696, -15.4905) -> (-34.4193, -15.4905)
  line L215 (-34.4193, -15.4905) -> (-34.4193, -12.2604)
  line L216 (-34.4193, -12.2604) -> (-35.2447, -12.2604)
  line L217 (-35.2447, -12.2604) -> (-35.2447, -9.4602)
  line L218 (-35.2447, -9.4602) -> (-34.4193, -9.4602)
  line L219 (-34.4193, -9.4602) -> (-34.4193, -3.1902)
  line L220 (-34.4193, -3.1902) -> (-32.694, -3.1902)
  line L221 (-32.694, -3.1902) -> (-32.694, -1.9899)
  line L222 (-32.694, -1.9899) -> (-29.3949, -1.9899)
  line L223 (-29.3949, -1.9899) -> (-29.3949, -3.1902)
  line L224 (-29.3949, -3.1902) -> (-27.6696, -3.1902)
  line L225 (-27.6696, -3.1902) -> (-27.6696, -7.6605)
  line L226 (-27.6696, -7.6605) -> (-26.9448, -7.6605)
  line L227 (-26.9448, -7.6605) -> (-26.9448, -3.5609)
  line L228 (-26.9448, -3.5609) -> (-26.1441, -3.5609)
  line L229 (-26.1441, -3.5609) -> (-26.1441, -2.96)
  line L230 (-26.1441, -2.96) -> (-12.1447, -2.96)
  line L231 (-12.1447, -2.96) -> (-12.1447, -3.5609)
  line L232 (-12.1447, -3.5609) -> (-11.344, -3.5609)
  line L233 (-11.344, -3.5609) -> (-11.344, -7.6605)
  line L234 (-11.344, -7.6605) -> (-10.6192, -7.6605)
  line L235 (-10.6192, -7.6605) -> (-10.6192, -3.1902)
  line L236 (-10.6192, -3.1902) -> (-8.8939, -3.1902)
  line L237 (-8.8939, -3.1902) -> (-8.8939, -1.9899)
  line L238 (-8.8939, -1.9899) -> (-5.5948, -1.9899)
  line L239 (-5.5948, -1.9899) -> (-5.5948, -3.1902)
  line L240 (-5.5948, -3.1902) -> (-3.8695, -3.1902)
  line L241 (-3.8695, -3.1902) -> (-3.8695, -9.4602)
  line L242 (-3.8695, -9.4602) -> (-3.0441, -9.4602)
  line L243 (-3.0441, -9.4602) -> (-3.0441, -12.2604)
  line L244 (-3.0441, -12.2604) -> (-3.8695, -12.2604)
  line L245 (-3.8695, -12.2604) -> (-3.8695, -15.4905)
  line L246 (-3.8695, -15.4905) -> (-10.6192, -15.4905)
  line L247 (-10.6192, -15.4905) -> (-10.6192, -12.2604)
  line L248 (-10.6192, -12.2604) -> (-11.344, -12.2604)
  line L249 (-11.344, -12.2604) -> (-11.344, -16.3601)
  line L250 (-11.344, -16.3601) -> (-12.1447, -16.3601)
  line L251 (-12.1447, -16.3601) -> (-12.1447, -16.9595)
  line L252 (-40.7197, -36.0094) -> (-54.719, -36.0094)
  line L253 (-54.719, -36.0094) -> (-54.719, -35.4101)
  line L254 (-54.719, -35.4101) -> (-55.5198, -35.4101)
  line L255 (-55.5198, -35.4101) -> (-55.5198, -22.6109)
  line L256 (-55.5198, -22.6109) -> (-54.719, -22.6109)
  line L257 (-54.719, -22.6109) -> (-54.719, -22.01)
  line L258 (-54.719, -22.01) -> (-40.7197, -22.01)
  line L259 (-40.7197, -22.01) -> (-40.7197, -22.6109)
  line L260 (-40.7197, -22.6109) -> (-39.9189, -22.6109)
  line L261 (-39.9189, -22.6109) -> (-39.9189, -35.4101)
  line L262 (-39.9189, -35.4101) -> (-40.7197, -35.4101)
  line L263 (-40.7197, -35.4101) -> (-40.7197, -36.0094)
  line L264 (-40.7197, -55.0594) -> (-54.719, -55.0594)
  line L265 (-54.719, -55.0594) -> (-54.719, -54.4601)
  line L266 (-54.719, -54.4601) -> (-55.5198, -54.4601)
  line L267 (-55.5198, -54.4601) -> (-55.5198, -41.6609)
  line L268 (-55.5198, -41.6609) -> (-54.719, -41.6609)
  line L269 (-54.719, -41.6609) -> (-54.719, -41.0602)
  line L270 (-54.719, -41.0602) -> (-40.7197, -41.0602)
  line L271 (-40.7197, -41.0602) -> (-40.7197, -41.6609)
  line L272 (-40.7197, -41.6609) -> (-39.9189, -41.6609)
  line L273 (-39.9189, -41.6609) -> (-39.9189, -54.4601)
  line L274 (-39.9189, -54.4601) -> (-40.7197, -54.4601)
  line L275 (-40.7197, -54.4601) -> (-40.7197, -55.0594)
  line L276 (-21.6697, -36.0094) -> (-35.669, -36.0094)
  line L277 (-35.669, -36.0094) -> (-35.669, -35.4101)
  line L278 (-35.669, -35.4101) -> (-36.4698, -35.4101)
  line L279 (-36.4698, -35.4101) -> (-36.4698, -22.6109)
  line L280 (-36.4698, -22.6109) -> (-35.669, -22.6109)
  line L281 (-35.669, -22.6109) -> (-35.669, -22.01)
  line L282 (-35.669, -22.01) -> (-21.6697, -22.01)
  line L283 (-21.6697, -22.01) -> (-21.6697, -22.6109)
  line L284 (-21.6697, -22.6109) -> (-20.869, -22.6109)
  line L285 (-20.869, -22.6109) -> (-20.869, -35.4101)
  line L286 (-20.869, -35.4101) -> (-21.6697, -35.4101)
  line L287 (-21.6697, -35.4101) -> (-21.6697, -36.0094)
  line L288 (-2.6197, -93.1594) -> (-16.6192, -93.1594)
  line L289 (-16.6192, -93.1594) -> (-16.6192, -92.5601)
  line L290 (-16.6192, -92.5601) -> (-17.4198, -92.5601)
  line L291 (-17.4198, -92.5601) -> (-17.4198, -79.7609)
  line L292 (-17.4198, -79.7609) -> (-16.6192, -79.7609)
  line L293 (-16.6192, -79.7609) -> (-16.6192, -79.1602)
  line L294 (-16.6192, -79.1602) -> (-2.6196, -79.1602)
  line L295 (-2.6197, -79.1602) -> (-2.6197, -79.7609)
  line L296 (-2.6197, -79.7609) -> (-1.819, -79.7609)
  line L297 (-1.819, -79.7609) -> (-1.819, -92.5601)
  line L298 (-1.819, -92.5601) -> (-2.6197, -92.5601)
  line L299 (-2.6197, -92.5601) -> (-2.6197, -93.1594)
  line L300 (-40.7197, -16.9595) -> (-54.719, -16.9595)
  line L301 (-54.719, -16.9595) -> (-54.719, -16.3601)
  line L302 (-54.719, -16.3601) -> (-55.5198, -16.3601)
  line L303 (-55.5198, -16.3601) -> (-55.5198, -3.5609)
  line L304 (-55.5198, -3.5609) -> (-54.719, -3.5609)
  line L305 (-54.719, -3.5609) -> (-54.719, -2.96)
  line L306 (-54.719, -2.96) -> (-40.7197, -2.96)
  line L307 (-40.7197, -2.96) -> (-40.7197, -3.5609)
  line L308 (-40.7197, -3.5609) -> (-39.9189, -3.5609)
  line L309 (-39.9189, -3.5609) -> (-39.9189, -16.3601)
  line L310 (-39.9189, -16.3601) -> (-40.7197, -16.3601)
  line L311 (-40.7197, -16.3601) -> (-40.7197, -16.9595)
  line L312 (-87.4343, -163.6) -> (11.1659, -163.6)
  line L313 (11.1659, -163.6) -> (11.1659, 14.2999)
  line L314 (11.1659, 14.2999) -> (-87.4343, 14.2999)
  line L315 (-87.4343, 14.2999) -> (-87.4343, -163.6)
  line L316 (16.1659, -163.6) -> (16.1659, -168.6)
  line L317 (16.1659, -168.6) -> (11.1659, -168.6)
  line L318 (-92.4343, 14.2999) -> (-92.4343, 19.2999)
  line L319 (-92.4343, 19.2999) -> (-87.4343, 19.2999)
  line L320 (-92.4343, 14.2999) -> (-92.4343, -168.6)
  line L321 (11.1659, -168.6) -> (-92.4343, -168.6)
  line L322 (16.1659, -163.6) -> (16.1659, 19.2999)
  line L323 (-87.4343, 19.2999) -> (16.1659, 19.2999)
  dimension "d53" = 5
  dimension "d54" = 5
  dimension "d55" = 5
  dimension "d56" = 5
  constraint vertical L316
  constraint horizontal L317
  constraint vertical L318
  constraint horizontal L319
  constraint perpendicular L312 L320
  constraint perpendicular L320 L321
  constraint perpendicular L314 L322
  constraint perpendicular L322 L323
  measures "d53" distance of L312.end L316.start
  measures "d54" distance of L312.end L317.end
  measures "d55" distance of L314.end L318.start
  measures "d56" distance of L314.end L319.end
extrude "Extrude21" add sketch "Sketch5" along normal blind 18 separate body contours L316 L317 L318 L319 L320 L321 L322 L323 makes body 3